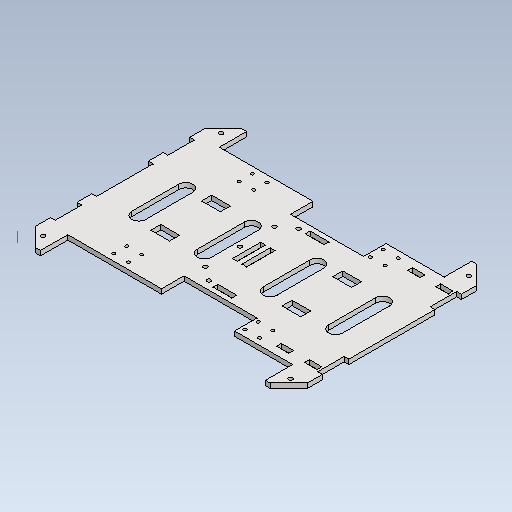
# Autodesk Inventor part: mid-plate
Saved by Autodesk Inventor 2025 (Build 290162000, 162)
## iProperties
Created: 2025-08-20
Part Number: mid-plate
Material: Generic
Document SubType Name: Modeling
Designer: HP
Density: 1 g/cm^3
Appearance: Default
Author: HP
Autodesk Inventor part; units mm, degrees
ref_plane "YZ Plane" through (0, 0, 0) normal (1, 0, 0) x (0, 1, 0)
ref_plane "XZ Plane" through (0, 0, 0) normal (0, 1, 0) x (-1, 0, 0)
ref_plane "XY Plane" through (0, 0, 0) normal (0, 0, 1) x (1, 0, 0)
sketch "Sketch1" plane through (0, 0, 0) normal (0, 1, 0) x (-1, 0, 0)
  line L0 (145, 110) -> (-145, 110)
  line L1 (-145, 110) -> (-145, -110)
  line L2 (-145, -110) -> (145, -110)
  line L3 (145, -110) -> (145, 110)
  line L4 (145, 110) -> (-145, -110) construction
  line L5 (-145, 110) -> (145, -110) construction
  line L6 (120, -80.8333) -> (20, -80.8333)
  line L7 (20, -80.8333) -> (20, -115.8333)
  line L8 (20, -115.8333) -> (120, -115.8333)
  line L9 (120, -115.8333) -> (120, -80.8333)
  line L10 (120, -80.8333) -> (20, -115.8333) construction
  line L11 (20, -80.8333) -> (120, -115.8333) construction
  line L12 (-20, -115.8333) -> (-120, -115.8333)
  line L13 (-120, -115.8333) -> (-120, -80.8333)
  line L14 (-120, -80.8333) -> (-20, -80.8333)
  line L15 (-20, -80.8333) -> (-20, -115.8333)
  line L16 (-20, -115.8333) -> (-120, -80.8333) construction
  line L17 (-120, -115.8333) -> (-20, -80.8333) construction
  line L18 (0, 110) -> (0, -110) construction
  point P0 (0, 0)
  point P1 (70, -98.3333)
  point P2 (-70, -98.3333)
  point P3 (0, 0)
  point P4 (-120, -110)
  point P5 (-20, -110)
  point P6 (120, -110)
  point P7 (20, -110)
  dimension "d1" = 100
  dimension "d2" = 100
  dimension "d3" = 35
  dimension "d4" = 35
  dimension "d5" = 140
  dimension "d6" = 11.6667
  dimension "d7" = 220
  dimension "d8" = 290
  constraints: 38 end point, 8 midpoint, 6 parallel, 3 horizontal, 3 perpendicular, 1 coincident, 1 horizontal alignment, 1 other
  measures "d1" distance between parallel lines of L7 L9
  measures "d2" distance between parallel lines of L13 L15
  measures "d3" distance between parallel lines of L6 L8
  measures "d4" distance between parallel lines of L14 L12
  measures "d5" distance of point (-70, -98.333) point (70, -98.333)
  measures "d6" distance from line of L2 point (70, -98.333)
  measures "d7" distance between parallel lines of L0 L2
  measures "d8" distance between parallel lines of L1 L3
extrude "Extrusion1" add sketch "Sketch1" along normal blind 5 contours L3 L2 L9 L6 L7 L15 L14 L13 L1 L0 | L2 L7 L6 L9 | L13 L14 L15 L2
extrude "Extrusion2" cut sketch "Sketch1" along normal blind 5 contours L9 L8 L7 L2 | L2 L7 L6 L9 | L13 L14 L15 L2
mirror "Mirror1" about plane through (0, 0, 0) normal (0, 0, 1) of "Extrusion2"
sketch "Sketch3" plane through (0, 5, 0) normal (0, 1, 0) x (1, 0, 0)
  line L0 (-120, -110) -> (-120, -80.8333) construction
  line L1 (-120, -80.8333) -> (-20, -80.8333) construction
  line L2 (-20, -80.8333) -> (-20, -110) construction
  line L3 (-20, -110) -> (20, -110) construction
  line L4 (20, -110) -> (20, -80.8333) construction
  line L5 (20, -80.8333) -> (120, -80.8333) construction
  line L6 (120, -80.8333) -> (120, -110) construction
  line L7 (120, -110) -> (145, -110) construction
  line L8 (145, -110) -> (145, 110) construction
  line L9 (145, 110) -> (120, 110) construction
  line L10 (120, 110) -> (120, 80.8333) construction
  line L11 (120, 80.8333) -> (20, 80.8333) construction
  line L12 (20, 80.8333) -> (20, 110) construction
  line L13 (20, 110) -> (-20, 110) construction
  line L14 (-20, 110) -> (-20, 80.8333) construction
  line L15 (-20, 80.8333) -> (-120, 80.8333) construction
  line L16 (-120, 80.8333) -> (-120, 110) construction
  line L17 (-120, 110) -> (-145, 110) projected
  line L18 (-145, 110) -> (-145, -110) construction
  line L19 (-145, -110) -> (-120, -110) construction
  circle A0 centre (-77.9, 73.7833) radius 1.6
  circle A1 centre (-62.1, 73.7833) radius 1.6
  circle A2 centre (-62.1, 59.8833) radius 1.6
  circle A3 centre (-77.9, 59.8833) radius 1.6
  line L20 (-77.9, 59.8833) -> (-62.1, 59.8833) construction
  line L21 (-62.1, 59.8833) -> (-62.1, 73.7833) construction
  line L22 (-62.1, 73.7833) -> (-77.9, 73.7833) construction
  line L23 (-77.9, 73.7833) -> (-77.9, 59.8833) construction
  line L24 (-77.9, 59.8833) -> (-62.1, 73.7833) construction
  line L25 (-62.1, 59.8833) -> (-77.9, 73.7833) construction
  point P0 (0, 0)
  point P1 (-70, 66.8333)
  point P2 (-70, 80.8333)
  dimension "d18" = 3.2
  dimension "d19" = 3.2
  dimension "d20" = 3.2
  dimension "d21" = 3.2
  dimension "d22" = 15.8
  dimension "d23" = 13.9
  dimension "d24" = 14
  constraints: 12 end point, 4 centre point, 4 coincident, 3 midpoint, 2 parallel, 1 horizontal, 1 perpendicular, 1 vertical alignment
  measures "d18" diameter of A0
  measures "d19" diameter of A1
  measures "d20" diameter of A3
  measures "d21" diameter of A2
  measures "d22" distance between parallel lines of L21 L23
  measures "d23" distance between parallel lines of L20 L22
  measures "d24" distance from line of point (-70, 66.833) L15
extrude "Extrusion4" cut sketch "Sketch3" against normal through all
mirror "Mirror4" about plane through (0, 0, 0) normal (1, 0, 0) of "Extrusion4"
mirror "Mirror5" about plane through (0, 0, 0) normal (0, 0, 1) of "Extrusion4", "Mirror4"
sketch "Sketch4" plane through (0, 5, 0) normal (0, 1, 0) x (1, 0, 0)
  circle A0 centre (62.1, -59.8833) radius 1.6 construction
  circle A1 centre (77.9, -59.8833) radius 1.6 construction
  circle A2 centre (62.1, -73.7833) radius 1.6 construction
  circle A3 centre (77.9, -73.7833) radius 1.6 construction
  circle A4 centre (-62.1, -59.8833) radius 1.6 construction
  circle A5 centre (-77.9, -59.8833) radius 1.6 construction
  circle A6 centre (-62.1, -73.7833) radius 1.6 construction
  circle A7 centre (-77.9, -73.7833) radius 1.6 construction
  circle A8 centre (62.1, 59.8833) radius 1.6 construction
  circle A9 centre (77.9, 59.8833) radius 1.6 construction
  circle A10 centre (62.1, 73.7833) radius 1.6 construction
  circle A11 centre (77.9, 73.7833) radius 1.6 construction
  circle A12 centre (-62.1, 59.8833) radius 1.6 construction
  circle A13 centre (-77.9, 73.7833) radius 1.6 construction
  circle A14 centre (-62.1, 73.7833) radius 1.6 construction
  circle A15 centre (-77.9, 59.8833) radius 1.6 construction
  line L0 (-120, -110) -> (-120, -80.8333) construction
  line L1 (-120, -80.8333) -> (-20, -80.8333) construction
  line L2 (-20, -80.8333) -> (-20, -110) construction
  line L3 (-20, -110) -> (20, -110) construction
  line L4 (20, -110) -> (20, -80.8333) construction
  line L5 (20, -80.8333) -> (120, -80.8333) construction
  line L6 (120, -80.8333) -> (120, -110) construction
  line L7 (120, -110) -> (145, -110) construction
  line L8 (145, -110) -> (145, 110) construction
  line L9 (145, 110) -> (120, 110) construction
  line L10 (120, 110) -> (120, 80.8333) construction
  line L11 (120, 80.8333) -> (20, 80.8333) construction
  line L12 (20, 80.8333) -> (20, 110) construction
  line L13 (20, 110) -> (-20, 110) construction
  line L14 (-20, 110) -> (-20, 80.8333) construction
  line L15 (-20, 80.8333) -> (-120, 80.8333) construction
  line L16 (-120, 80.8333) -> (-120, 110) construction
  line L17 (-120, 110) -> (-145, 110) construction
  line L18 (-145, 110) -> (-145, -110) construction
  line L19 (-145, -110) -> (-120, -110) construction
  line L20 (65, 17.6333) -> (45, 17.6333)
  line L21 (45, 17.6333) -> (45, 20.8333)
  line L22 (45, 20.8333) -> (65, 20.8333)
  line L23 (65, 20.8333) -> (65, 17.6333)
  line L24 (65, 17.6333) -> (45, 20.8333) construction
  line L25 (45, 17.6333) -> (65, 20.8333) construction
  point P0 (0, 0)
  point P1 (55, 19.2333)
  dimension "d27" = 20
  dimension "d28" = 3.2
  dimension "d29" = 80
  dimension "d30" = 60
  constraints: 12 end point, 2 midpoint, 2 parallel, 1 horizontal, 1 perpendicular
  measures "d27" distance between parallel lines of L23 L21
  measures "d28" distance between parallel lines of L22 L20
  measures "d29" distance between parallel lines of L8 L23
  measures "d30" distance between parallel lines of L11 L22
extrude "Extrusion5" [suppressed]
sketch "Sketch5" plane through (0, 5, 0) normal (0, 1, 0) x (1, 0, 0)
  circle A0 centre (62.1, -59.8833) radius 1.6 construction
  circle A1 centre (77.9, -59.8833) radius 1.6 construction
  circle A2 centre (62.1, -73.7833) radius 1.6 construction
  circle A3 centre (77.9, -73.7833) radius 1.6 construction
  circle A4 centre (-62.1, -59.8833) radius 1.6 construction
  circle A5 centre (-77.9, -59.8833) radius 1.6 construction
  circle A6 centre (-62.1, -73.7833) radius 1.6 construction
  circle A7 centre (-77.9, -73.7833) radius 1.6 construction
  circle A8 centre (62.1, 59.8833) radius 1.6 construction
  circle A9 centre (77.9, 59.8833) radius 1.6 construction
  circle A10 centre (62.1, 73.7833) radius 1.6 construction
  circle A11 centre (77.9, 73.7833) radius 1.6 construction
  circle A12 centre (-62.1, 59.8833) radius 1.6 construction
  circle A13 centre (-77.9, 73.7833) radius 1.6 construction
  circle A14 centre (-62.1, 73.7833) radius 1.6 construction
  circle A15 centre (-77.9, 59.8833) radius 1.6 construction
  line L0 (-120, -110) -> (-120, -80.8333) construction
  line L1 (-120, -80.8333) -> (-20, -80.8333) construction
  line L2 (-20, -80.8333) -> (-20, -110) projected
  line L3 (-20, -110) -> (20, -110) projected
  line L4 (20, -110) -> (20, -80.8333) projected
  line L5 (20, -80.8333) -> (120, -80.8333) construction
  line L6 (120, -80.8333) -> (120, -110) construction
  line L7 (120, -110) -> (145, -110) construction
  line L8 (145, -110) -> (145, 110) construction
  line L9 (145, 110) -> (120, 110) construction
  line L10 (120, 110) -> (120, 80.8333) construction
  line L11 (120, 80.8333) -> (20, 80.8333) construction
  line L12 (20, 80.8333) -> (20, 110) construction
  line L13 (20, 110) -> (-20, 110) construction
  line L14 (-20, 110) -> (-20, 80.8333) construction
  line L15 (-20, 80.8333) -> (-120, 80.8333) construction
  line L16 (-120, 80.8333) -> (-120, 110) construction
  line L17 (-120, 110) -> (-145, 110) construction
  line L18 (-145, 110) -> (-145, -110) construction
  line L19 (-145, -110) -> (-120, -110) construction
  line L20 (-20, -80.8333) -> (52, -80.8333)
  line L21 (52, -80.8333) -> (52, -56.8333)
  line L22 (52, -56.8333) -> (-20, -56.8333)
  line L23 (-20, -56.8333) -> (-20, -80.8333)
  line L24 (-20, -80.8333) -> (52, -56.8333) construction
  line L25 (52, -80.8333) -> (-20, -56.8333) construction
  line L26 (-20, -80.8333) -> (-20, -110) construction
  line L27 (124.4, -72.6) -> (137.6, -72.6)
  line L28 (137.6, -72.6) -> (137.6, -67.4)
  line L29 (137.6, -67.4) -> (124.4, -67.4)
  line L30 (124.4, -67.4) -> (124.4, -72.6)
  line L31 (124.4, -72.6) -> (137.6, -67.4) construction
  line L32 (137.6, -72.6) -> (124.4, -67.4) construction
  line L33 (26.1, -51.8333) -> (5.9, -51.8333)
  line L34 (5.9, -51.8333) -> (5.9, -46.6333)
  line L35 (5.9, -46.6333) -> (26.1, -46.6333)
  line L36 (26.1, -46.6333) -> (26.1, -51.8333)
  line L37 (26.1, -51.8333) -> (5.9, -46.6333) construction
  line L38 (5.9, -51.8333) -> (26.1, -46.6333) construction
  line L39 (60.2, -21.7333) -> (80.2, -21.7333)
  line L40 (80.2, -21.7333) -> (80.2, -32.4333)
  line L41 (80.2, -32.4333) -> (60.2, -32.4333)
  line L42 (60.2, -32.4333) -> (60.2, -21.7333)
  line L43 (60.2, -21.7333) -> (80.2, -32.4333) construction
  line L44 (80.2, -21.7333) -> (60.2, -32.4333) construction
  line L45 (-79.8, -32.4333) -> (-59.8, -32.4333)
  line L46 (-59.8, -32.4333) -> (-59.8, -21.7333)
  line L47 (-59.8, -21.7333) -> (-79.8, -21.7333)
  line L48 (-79.8, -21.7333) -> (-79.8, -32.4333)
  line L49 (-79.8, -32.4333) -> (-59.8, -21.7333) construction
  line L50 (-59.8, -32.4333) -> (-79.8, -21.7333) construction
  line L51 (52, -56.8333) -> (58, -56.8333)
  line L52 (58, -56.8333) -> (58, -80.8333)
  line L53 (58, -80.8333) -> (52, -80.8333)
  line L54 (52, -80.8333) -> (52, -56.8333)
  line L55 (94.4, -72.6) -> (107.6, -72.6)
  line L56 (107.6, -72.6) -> (107.6, -67.4)
  line L57 (107.6, -67.4) -> (94.4, -67.4)
  line L58 (94.4, -67.4) -> (94.4, -72.6)
  line L59 (94.4, -72.6) -> (107.6, -67.4) construction
  line L60 (107.6, -72.6) -> (94.4, -67.4) construction
  point P0 (0, 0)
  point P1 (16, -68.8333)
  point P2 (20, -80.8333)
  point P3 (131, -70)
  point P4 (131, -72.6)
  point P5 (16, -49.2333)
  point P6 (70.2, -27.0833)
  point P7 (-69.8, -27.0833)
  point P8 (52, -80.8333)
  point P9 (52, -80.8333)
  point P10 (101, -70)
  point P11 (101, -72.6)
  dimension "d33" = 24
  dimension "d34" = 72
  dimension "d37" = 13.2
  dimension "d38" = 5.2
  dimension "d40" = 14
  dimension "d55" = 20.2
  dimension "d56" = 5.2
  dimension "d57" = 5
  dimension "d60" = 20
  dimension "d61" = 10.7
  dimension "d62" = 53.75
  dimension "d63" = 74.8
  dimension "d64" = 75.2
  dimension "d65" = 10.7
  dimension "d66" = 20
  dimension "d85" = 6
  dimension "d105" = 70
  dimension "d106" = 13.2
  dimension "d107" = 5.2
  dimension "d108" = 30
  constraints: 80 end point, 14 midpoint, 14 parallel, 7 horizontal, 7 perpendicular, 2 collinear, 2 horizontal alignment, 1 point on line, 1 vertical alignment
  measures "d33" distance between parallel lines of L22 L20
  measures "d34" distance between parallel lines of L21 L23
  measures "d37" distance between parallel lines of L28 L30
  measures "d38" distance between parallel lines of L27 L29
  measures "d40" distance from line of L8 point (131, -72.6)
  measures "d55" distance of L34.end L35.end
  measures "d56" distance between parallel lines of L35 L33
  measures "d57" distance between parallel lines of L33 L22
  measures "d60" distance between parallel lines of L40 L42
  measures "d61" distance between parallel lines of L41 L39
  measures "d62" distance from line of point (70.2, -27.083) L5
  measures "d63" distance from line of L8 point (70.2, -27.083)
  measures "d64" distance from line of L18 point (-69.8, -27.083)
  measures "d65" distance between parallel lines of L45 L47
  measures "d66" distance between parallel lines of L46 L48
  measures "d85" distance between parallel lines of L52 L54
  measures "d105" vertical distance of point (131, -70) point (0, 0)
  measures "d106" distance between parallel lines of L56 L58
  measures "d107" distance between parallel lines of L55 L57
  measures "d108" distance of point (131, -70) point (101, -70)
extrude "Extrusion6" cut sketch "Sketch5" against normal through all
mirror "Mirror6" about plane through (0, 0, 0) normal (0, 0, 1) of "Extrusion6"
sketch "Sketch6" plane through (0, 5, 0) normal (0, 1, 0) x (1, 0, 0)
  circle A0 centre (-77.9, 59.8833) radius 1.6 construction
  circle A1 centre (-62.1, 73.7833) radius 1.6 construction
  circle A2 centre (-77.9, 73.7833) radius 1.6 construction
  circle A3 centre (-62.1, 59.8833) radius 1.6 construction
  circle A4 centre (77.9, 73.7833) radius 1.6 construction
  circle A5 centre (62.1, 73.7833) radius 1.6 construction
  circle A6 centre (77.9, 59.8833) radius 1.6 construction
  circle A7 centre (62.1, 59.8833) radius 1.6 construction
  circle A8 centre (-77.9, -73.7833) radius 1.6 construction
  circle A9 centre (-62.1, -73.7833) radius 1.6 construction
  circle A10 centre (-77.9, -59.8833) radius 1.6 construction
  circle A11 centre (-62.1, -59.8833) radius 1.6 construction
  circle A12 centre (77.9, -73.7833) radius 1.6 construction
  circle A13 centre (62.1, -73.7833) radius 1.6 construction
  circle A14 centre (77.9, -59.8833) radius 1.6 construction
  circle A15 centre (62.1, -59.8833) radius 1.6 construction
  line L0 (124.4, -67.4) -> (137.6, -67.4) construction
  line L1 (137.6, -67.4) -> (137.6, -72.6) construction
  line L2 (137.6, -72.6) -> (124.4, -72.6) construction
  line L3 (124.4, -72.6) -> (124.4, -67.4) construction
  line L4 (-20, 56.8333) -> (-20, 80.8333) construction
  line L5 (-20, 80.8333) -> (-120, 80.8333) construction
  line L6 (-120, 80.8333) -> (-120, 110) construction
  line L7 (-120, 110) -> (-145, 110) construction
  line L8 (-145, 110) -> (-145, -110) construction
  line L9 (-145, -110) -> (-120, -110) construction
  line L10 (-120, -110) -> (-120, -80.8333) construction
  line L11 (-120, -80.8333) -> (-20, -80.8333) construction
  line L12 (-20, -80.8333) -> (-20, -56.8333) construction
  line L13 (58, -80.8333) -> (120, -80.8333) construction
  line L14 (120, -80.8333) -> (120, -110) construction
  line L15 (120, -110) -> (145, -110) construction
  line L16 (145, -110) -> (145, 110) construction
  line L17 (145, 110) -> (120, 110) construction
  line L18 (120, 110) -> (120, 80.8333) construction
  line L19 (120, 80.8333) -> (58, 80.8333) construction
  line L20 (124.4, 67.4) -> (124.4, 72.6) construction
  line L21 (124.4, 72.6) -> (137.6, 72.6) construction
  line L22 (137.6, 72.6) -> (137.6, 67.4) construction
  line L23 (137.6, 67.4) -> (124.4, 67.4) construction
  line L24 (-140, 30.1) -> (-145, 30.1)
  line L25 (-145, 30.1) -> (-145, -30.1)
  line L26 (-145, -30.1) -> (-140, -30.1)
  line L27 (-140, -30.1) -> (-140, 30.1)
  line L28 (-140, 30.1) -> (-145, -30.1) construction
  line L29 (-145, 30.1) -> (-140, -30.1) construction
  line L30 (-145, 110) -> (-145, -110) projected
  line L31 (-10.1, 15.1) -> (-4.9, 15.1)
  line L32 (-4.9, 15.1) -> (-4.9, -15.1)
  line L33 (-4.9, -15.1) -> (-10.1, -15.1)
  line L34 (-10.1, -15.1) -> (-10.1, 15.1)
  line L35 (-10.1, 15.1) -> (-4.9, -15.1) construction
  line L36 (-4.9, 15.1) -> (-10.1, -15.1) construction
  line L37 (5.3, -15.1) -> (0.1, -15.1)
  line L38 (0.1, -15.1) -> (0.1, 15.1)
  line L39 (0.1, 15.1) -> (5.3, 15.1)
  line L40 (5.3, 15.1) -> (5.3, -15.1)
  line L41 (5.3, -15.1) -> (0.1, 15.1) construction
  line L42 (0.1, -15.1) -> (5.3, 15.1) construction
  line L43 (-100, 25) -> (-100, -25) construction
  line L44 (-107.5, 25) -> (-107.5, -25)
  line L45 (-92.5, -25) -> (-92.5, 25)
  arc A16 (-92.5, 25) -> (-107.5, 25) centre (-100, 25) ccw
  arc A17 (-107.5, -25) -> (-92.5, -25) centre (-100, -25) ccw
  line L46 (-30, 25) -> (-30, -25) construction
  line L47 (-37.5, 25) -> (-37.5, -25)
  line L48 (-22.5, -25) -> (-22.5, 25)
  arc A18 (-22.5, 25) -> (-37.5, 25) centre (-30, 25) ccw
  arc A19 (-37.5, -25) -> (-22.5, -25) centre (-30, -25) ccw
  line L49 (40, 25) -> (40, -25) construction
  line L50 (32.5, 25) -> (32.5, -25)
  line L51 (47.5, -25) -> (47.5, 25)
  arc A20 (47.5, 25) -> (32.5, 25) centre (40, 25) ccw
  arc A21 (32.5, -25) -> (47.5, -25) centre (40, -25) ccw
  line L52 (110, 25) -> (110, -25) construction
  line L53 (102.5, 25) -> (102.5, -25)
  line L54 (117.5, -25) -> (117.5, 25)
  arc A22 (117.5, 25) -> (102.5, 25) centre (110, 25) ccw
  arc A23 (102.5, -25) -> (117.5, -25) centre (110, -25) ccw
  line L55 (-20, -56.8333) -> (58, -56.8333) projected
  line L56 (58, -56.8333) -> (58, -80.8333) projected
  line L57 (58, 80.8333) -> (58, 56.8333) projected
  line L58 (58, 56.8333) -> (-20, 56.8333) projected
  point P0 (0, 0)
  point P1 (-142.5, 0)
  point P2 (-145, 0)
  point P3 (-7.5, 0)
  point P4 (2.7, 0)
  point P5 (-100, 0)
  point P6 (-30, 0)
  point P7 (40, 0)
  point P8 (110, 0)
  point P9 (-145, 0)
  dimension "d41" = 60.2
  dimension "d42" = 5
  dimension "d49" = 5.2
  dimension "d50" = 30.2
  dimension "d51" = 134.9
  dimension "d52" = 5.2
  dimension "d53" = 30.2
  dimension "d67" = 15
  dimension "d68" = 15
  dimension "d69" = 15
  dimension "d70" = 15
  dimension "d71" = 50
  dimension "d72" = 50
  dimension "d73" = 50
  dimension "d74" = 50
  dimension "d75" = 45
  dimension "d76" = 115
  dimension "d77" = 105
  dimension "d78" = 35
  dimension "d109" = 10.2
  constraints: 68 end point, 16 point on circle, 16 tangent, 13 parallel, 12 midpoint, 8 centre point, 7 horizontal alignment, 3 horizontal, 3 perpendicular, 1 collinear, 1 vertical
  measures "d41" distance between parallel lines of L26 L24
  measures "d42" distance between parallel lines of L8 L27
  measures "d49" distance of L32.end L33.end
  measures "d50" distance of L31.end L32.end
  measures "d51" distance between parallel lines of L8 L34
  measures "d52" distance between parallel lines of L38 L40
  measures "d53" distance between parallel lines of L39 L37
  measures "d67" distance between parallel lines of L51 L50
  measures "d68" distance between parallel lines of L45 L44
  measures "d69" distance between parallel lines of L48 L47
  measures "d70" distance between parallel lines of L54 L53
  measures "d71" distance of L52.start L52.end
  measures "d72" distance of L43.start L43.end
  measures "d73" distance of L46.start L46.end
  measures "d74" distance of L49.start L49.end
  measures "d75" distance from line of L8 point (-100, 0)
  measures "d76" distance from line of L8 point (-30, 0)
  measures "d77" distance from line of L16 point (40, 0)
  measures "d78" distance from line of L16 point (110, 0)
  measures "d109" distance of point (2.7, 0) point (-7.5, 0)
extrude "Extrusion7" cut sketch "Sketch6" against normal through all
chamfer "Chamfer1" distance 20 angle 45 4 edges at (-145, 2.5, 110) (-145, 2.5, -110) (145, 2.5, 110) (145, 2.5, -110)
sketch "Sketch8" plane through (0, 5, 0) normal (0, 1, 0) x (1, 0, 0)
  line L0 (125, 110) -> (145, 90) construction
  line L1 (125, 110) -> (120, 110) construction
  line L2 (120, 110) -> (120, 80.8333) construction
  line L3 (120, 80.8333) -> (58, 80.8333) construction
  line L4 (-20, 56.8333) -> (-20, 80.8333) construction
  line L5 (-20, 80.8333) -> (-120, 80.8333) construction
  line L6 (-120, 80.8333) -> (-120, 110) construction
  line L7 (-120, 110) -> (-125, 110) construction
  line L8 (-145, 90) -> (-125, 110) construction
  line L9 (-145, 90) -> (-145, 30.1) projected
  line L10 (-145, 30.1) -> (-140, 30.1) construction
  line L11 (-140, 30.1) -> (-140, -30.1) construction
  line L12 (-140, -30.1) -> (-145, -30.1) construction
  line L13 (-145, -30.1) -> (-145, -90) construction
  line L14 (-125, -110) -> (-145, -90) construction
  line L15 (-125, -110) -> (-120, -110) construction
  line L16 (-120, -110) -> (-120, -80.8333) construction
  line L17 (-120, -80.8333) -> (-20, -80.8333) construction
  line L18 (-20, -80.8333) -> (-20, -56.8333) construction
  line L19 (58, -80.8333) -> (120, -80.8333) construction
  line L20 (120, -80.8333) -> (120, -110) construction
  line L21 (120, -110) -> (125, -110) construction
  line L22 (145, -90) -> (125, -110) construction
  line L23 (145, -90) -> (145, 90) construction
  line L24 (124.4, -67.4) -> (137.6, -67.4) construction
  line L25 (137.6, -67.4) -> (137.6, -72.6) construction
  line L26 (137.6, -72.6) -> (124.4, -72.6) construction
  line L27 (124.4, -72.6) -> (124.4, -67.4) construction
  line L28 (5.9, -51.8333) -> (5.9, -46.6333) construction
  line L29 (5.9, -46.6333) -> (26.1, -46.6333) construction
  line L30 (26.1, -46.6333) -> (26.1, -51.8333) construction
  line L31 (26.1, -51.8333) -> (5.9, -51.8333) construction
  line L32 (80.2, -21.7333) -> (80.2, -32.4333) construction
  line L33 (80.2, -32.4333) -> (60.2, -32.4333) construction
  line L34 (60.2, -32.4333) -> (60.2, -21.7333) construction
  line L35 (60.2, -21.7333) -> (80.2, -21.7333) construction
  line L36 (-79.8, -21.7333) -> (-59.8, -21.7333) construction
  line L37 (-59.8, -21.7333) -> (-59.8, -32.4333) construction
  line L38 (-59.8, -32.4333) -> (-79.8, -32.4333) construction
  line L39 (-79.8, -32.4333) -> (-79.8, -21.7333) construction
  circle A0 centre (62.1, -59.8833) radius 1.6 construction
  circle A1 centre (77.9, -59.8833) radius 1.6 construction
  circle A2 centre (62.1, -73.7833) radius 1.6 construction
  circle A3 centre (77.9, -73.7833) radius 1.6 construction
  circle A4 centre (-62.1, -59.8833) radius 1.6 construction
  circle A5 centre (-77.9, -59.8833) radius 1.6 construction
  circle A6 centre (-62.1, -73.7833) radius 1.6 construction
  circle A7 centre (-77.9, -73.7833) radius 1.6 construction
  circle A8 centre (62.1, 59.8833) radius 1.6 construction
  circle A9 centre (77.9, 59.8833) radius 1.6 construction
  circle A10 centre (62.1, 73.7833) radius 1.6 construction
  circle A11 centre (77.9, 73.7833) radius 1.6 construction
  circle A12 centre (-62.1, 59.8833) radius 1.6 construction
  circle A13 centre (-77.9, 73.7833) radius 1.6 construction
  circle A14 centre (-62.1, 73.7833) radius 1.6 construction
  circle A15 centre (-77.9, 59.8833) radius 1.6 construction
  line L40 (26.1, 51.8333) -> (26.1, 46.6333) construction
  line L41 (26.1, 46.6333) -> (5.9, 46.6333) construction
  line L42 (5.9, 46.6333) -> (5.9, 51.8333) construction
  line L43 (5.9, 51.8333) -> (26.1, 51.8333) construction
  line L44 (80.2, 21.7333) -> (60.2, 21.7333) construction
  line L45 (60.2, 21.7333) -> (60.2, 32.4333) construction
  line L46 (60.2, 32.4333) -> (80.2, 32.4333) construction
  line L47 (80.2, 32.4333) -> (80.2, 21.7333) construction
  line L48 (-79.8, 32.4333) -> (-59.8, 32.4333) construction
  line L49 (-59.8, 32.4333) -> (-59.8, 21.7333) construction
  line L50 (-59.8, 21.7333) -> (-79.8, 21.7333) construction
  line L51 (-79.8, 21.7333) -> (-79.8, 32.4333) construction
  line L52 (124.4, 72.6) -> (137.6, 72.6) construction
  line L53 (137.6, 72.6) -> (137.6, 67.4) construction
  line L54 (137.6, 67.4) -> (124.4, 67.4) construction
  line L55 (124.4, 67.4) -> (124.4, 72.6) construction
  line L56 (-4.9, 15.1) -> (-4.9, -15.1) construction
  line L57 (-4.9, -15.1) -> (-10.1, -15.1) construction
  line L58 (-10.1, -15.1) -> (-10.1, 15.1) construction
  line L59 (-10.1, 15.1) -> (-4.9, 15.1) construction
  line L60 (-22.5, 25) -> (-22.5, -25) construction
  arc A16 (-37.5, -25) -> (-22.5, -25) centre (-30, -25) ccw construction
  line L61 (-37.5, -25) -> (-37.5, 25) construction
  arc A17 (-22.5, 25) -> (-37.5, 25) centre (-30, 25) ccw construction
  line L62 (-92.5, 25) -> (-92.5, -25) construction
  arc A18 (-107.5, -25) -> (-92.5, -25) centre (-100, -25) ccw construction
  line L63 (-107.5, -25) -> (-107.5, 25) construction
  arc A19 (-92.5, 25) -> (-107.5, 25) centre (-100, 25) ccw construction
  line L64 (117.5, 25) -> (117.5, -25) construction
  arc A20 (102.5, -25) -> (117.5, -25) centre (110, -25) ccw construction
  line L65 (102.5, -25) -> (102.5, 25) construction
  arc A21 (117.5, 25) -> (102.5, 25) centre (110, 25) ccw construction
  line L66 (0.1, -15.1) -> (0.1, 15.1) construction
  line L67 (0.1, 15.1) -> (5.3, 15.1) construction
  line L68 (5.3, 15.1) -> (5.3, -15.1) construction
  line L69 (5.3, -15.1) -> (0.1, -15.1) construction
  line L70 (47.5, 25) -> (47.5, -25) construction
  arc A22 (32.5, -25) -> (47.5, -25) centre (40, -25) ccw construction
  line L71 (32.5, -25) -> (32.5, 25) construction
  arc A23 (47.5, 25) -> (32.5, 25) centre (40, 25) ccw construction
  circle A24 centre (-2.4, -48) radius 2.1
  line L72 (-4.9, -15.1) -> (0.1, -15.1) construction
  circle A25 centre (-2.4, 48) radius 2.1
  line L73 (58, 80.8333) -> (58, 56.8333) projected
  line L74 (58, 56.8333) -> (-20, 56.8333) projected
  line L75 (-20, -56.8333) -> (58, -56.8333) projected
  line L76 (58, -56.8333) -> (58, -80.8333) projected
  line L77 (-145, 45.95) -> (-140, 45.95)
  line L78 (-140, 45.95) -> (-140, 74.15)
  line L79 (-140, 74.15) -> (-145, 74.15)
  line L80 (-145, 74.15) -> (-145, 45.95)
  line L81 (-145, 45.95) -> (-140, 74.15) construction
  line L82 (-140, 45.95) -> (-145, 74.15) construction
  line L83 (-145, 90) -> (-145, 30.1) projected
  line L84 (-145, -45.95) -> (-140, -45.95)
  line L85 (-140, -45.95) -> (-140, -74.15)
  line L86 (-140, -74.15) -> (-145, -74.15)
  line L87 (-145, -74.15) -> (-145, -45.95)
  line L88 (-145, -45.95) -> (-140, -74.15) construction
  line L89 (-140, -45.95) -> (-145, -74.15) construction
  line L90 (140, 74.15) -> (145, 74.15)
  line L91 (145, 74.15) -> (145, 45.95)
  line L92 (145, 45.95) -> (140, 45.95)
  line L93 (140, 45.95) -> (140, 74.15)
  line L94 (140, 74.15) -> (145, 45.95) construction
  line L95 (145, 74.15) -> (140, 45.95) construction
  line L96 (140, -45.95) -> (145, -45.95)
  line L97 (145, -45.95) -> (145, -74.15)
  line L98 (145, -74.15) -> (140, -74.15)
  line L99 (140, -74.15) -> (140, -45.95)
  line L100 (140, -45.95) -> (145, -74.15) construction
  line L101 (145, -45.95) -> (140, -74.15) construction
  line L102 (145, -90) -> (145, 90) construction
  circle A26 centre (-17.1, -37) radius 2.1
  circle A27 centre (-17.1, 0) radius 2.1
  circle A28 centre (-17.1, 37) radius 2.1
  point P0 (0, 0)
  point P1 (-2.4, -15.1)
  point P2 (-142.5, 60.05)
  point P3 (-145, 60.05)
  point P4 (-142.5, -60.05)
  point P5 (-145, -60.05)
  point P6 (142.5, 60.05)
  point P7 (142.5, -60.05)
  point P8 (0.1, 0)
  dimension "d79" = 4.2
  dimension "d80" = 4.2
  dimension "d88" = 5
  dimension "d89" = 28.2
  dimension "d91" = 28.2
  dimension "d92" = 5
  dimension "d93" = 28.2
  dimension "d94" = 28.2
  dimension "d95" = 5
  dimension "d96" = 5
  dimension "d110" = 4.2
  dimension "d111" = 4.2
  dimension "d112" = 4.2
  dimension "d113" = 37
  dimension "d114" = 37
  dimension "d115" = 7
  dimension "d116" = 48
  dimension "d117" = 48
  constraints: 50 end point, 12 midpoint, 8 parallel, 5 centre point, 5 horizontal, 5 horizontal alignment, 5 vertical alignment, 4 perpendicular, 3 collinear
  measures "d79" diameter of A24
  measures "d80" diameter of A25
  measures "d88" distance between parallel lines of L80 L78
  measures "d89" distance between parallel lines of L77 L79
  measures "d91" distance between parallel lines of L86 L84
  measures "d92" distance between parallel lines of L87 L85
  measures "d93" distance between parallel lines of L98 L96
  measures "d94" distance between parallel lines of L92 L90
  measures "d95" distance between parallel lines of L91 L93
  measures "d96" distance between parallel lines of L23 L99
  measures "d110" diameter of A26
  measures "d111" diameter of A27
  measures "d112" diameter of A28
  measures "d113" distance of A27.centre A28.centre
  measures "d114" distance of A26.centre A27.centre
  measures "d115" distance from line of A27.centre L58
  measures "d116" vertical distance of point (0, 0) A25.centre
  measures "d117" vertical distance of A24.centre point (0, 0)
extrude "Extrusion8" cut sketch "Sketch8" against normal through all
sketch "Sketch9" plane through (0, 5, 0) normal (0, 1, 0) x (1, 0, 0)
  line L0 (47.5, 25) -> (47.5, -25) construction
  arc A0 (32.5, -25) -> (47.5, -25) centre (40, -25) ccw construction
  line L1 (32.5, -25) -> (32.5, 25) construction
  arc A1 (47.5, 25) -> (32.5, 25) centre (40, 25) ccw construction
  line L2 (0.1, -15.1) -> (0.1, 15.1) construction
  line L3 (0.1, 15.1) -> (5.3, 15.1) construction
  line L4 (5.3, 15.1) -> (5.3, -15.1) construction
  line L5 (5.3, -15.1) -> (0.1, -15.1) construction
  line L6 (117.5, 25) -> (117.5, -25) construction
  arc A2 (102.5, -25) -> (117.5, -25) centre (110, -25) ccw construction
  line L7 (102.5, -25) -> (102.5, 25) construction
  arc A3 (117.5, 25) -> (102.5, 25) centre (110, 25) ccw construction
  line L8 (-92.5, 25) -> (-92.5, -25) construction
  arc A4 (-107.5, -25) -> (-92.5, -25) centre (-100, -25) ccw construction
  line L9 (-107.5, -25) -> (-107.5, 25) construction
  arc A5 (-92.5, 25) -> (-107.5, 25) centre (-100, 25) ccw construction
  line L10 (-22.5, 25) -> (-22.5, -25) construction
  arc A6 (-37.5, -25) -> (-22.5, -25) centre (-30, -25) ccw construction
  line L11 (-37.5, -25) -> (-37.5, 25) construction
  arc A7 (-22.5, 25) -> (-37.5, 25) centre (-30, 25) ccw construction
  line L12 (-4.9, 15.1) -> (-4.9, -15.1) construction
  line L13 (-4.9, -15.1) -> (-10.1, -15.1) construction
  line L14 (-10.1, -15.1) -> (-10.1, 15.1) construction
  line L15 (-10.1, 15.1) -> (-4.9, 15.1) construction
  line L16 (26.1, 51.8333) -> (26.1, 46.6333) construction
  line L17 (26.1, 46.6333) -> (5.9, 46.6333) construction
  line L18 (5.9, 46.6333) -> (5.9, 51.8333) construction
  line L19 (5.9, 51.8333) -> (26.1, 51.8333) construction
  line L20 (60.2, 21.7333) -> (60.2, 32.4333) construction
  line L21 (60.2, 32.4333) -> (80.2, 32.4333) construction
  line L22 (80.2, 32.4333) -> (80.2, 21.7333) construction
  line L23 (80.2, 21.7333) -> (60.2, 21.7333) construction
  line L24 (-79.8, 21.7333) -> (-79.8, 32.4333) construction
  line L25 (-79.8, 32.4333) -> (-59.8, 32.4333) construction
  line L26 (-59.8, 32.4333) -> (-59.8, 21.7333) construction
  line L27 (-59.8, 21.7333) -> (-79.8, 21.7333) construction
  line L28 (124.4, 72.6) -> (137.6, 72.6) construction
  line L29 (137.6, 72.6) -> (137.6, 67.4) construction
  line L30 (137.6, 67.4) -> (124.4, 67.4) construction
  line L31 (124.4, 67.4) -> (124.4, 72.6) construction
  circle A8 centre (-77.9, 59.8833) radius 1.6 construction
  circle A9 centre (-62.1, 73.7833) radius 1.6 construction
  circle A10 centre (-77.9, 73.7833) radius 1.6 construction
  circle A11 centre (-62.1, 59.8833) radius 1.6 construction
  circle A12 centre (77.9, 73.7833) radius 1.6 construction
  circle A13 centre (62.1, 73.7833) radius 1.6 construction
  circle A14 centre (77.9, 59.8833) radius 1.6 construction
  circle A15 centre (62.1, 59.8833) radius 1.6 construction
  circle A16 centre (-77.9, -73.7833) radius 1.6 construction
  circle A17 centre (-62.1, -73.7833) radius 1.6 construction
  circle A18 centre (-77.9, -59.8833) radius 1.6 construction
  circle A19 centre (-62.1, -59.8833) radius 1.6 construction
  circle A20 centre (77.9, -73.7833) radius 1.6 construction
  circle A21 centre (62.1, -73.7833) radius 1.6 construction
  circle A22 centre (77.9, -59.8833) radius 1.6 construction
  circle A23 centre (62.1, -59.8833) radius 1.6 construction
  line L32 (80.2, -21.7333) -> (80.2, -32.4333) construction
  line L33 (80.2, -32.4333) -> (60.2, -32.4333) construction
  line L34 (60.2, -32.4333) -> (60.2, -21.7333) construction
  line L35 (60.2, -21.7333) -> (80.2, -21.7333) construction
  line L36 (-79.8, -21.7333) -> (-59.8, -21.7333) construction
  line L37 (-59.8, -21.7333) -> (-59.8, -32.4333) construction
  line L38 (-59.8, -32.4333) -> (-79.8, -32.4333) construction
  line L39 (-79.8, -32.4333) -> (-79.8, -21.7333) construction
  line L40 (124.4, -67.4) -> (137.6, -67.4) construction
  line L41 (137.6, -67.4) -> (137.6, -72.6) construction
  line L42 (137.6, -72.6) -> (124.4, -72.6) construction
  line L43 (124.4, -72.6) -> (124.4, -67.4) construction
  line L44 (5.9, -51.8333) -> (5.9, -46.6333) construction
  line L45 (5.9, -46.6333) -> (26.1, -46.6333) construction
  line L46 (26.1, -46.6333) -> (26.1, -51.8333) construction
  line L47 (26.1, -51.8333) -> (5.9, -51.8333) construction
  circle A24 centre (-2.4, 48) radius 2.1 construction
  circle A25 centre (-2.4, -48) radius 2.1 construction
  line L48 (-145, 74.15) -> (-140, 74.15) construction
  line L49 (-140, 74.15) -> (-140, 45.95) construction
  line L50 (-140, 45.95) -> (-145, 45.95) construction
  line L51 (-145, 45.95) -> (-145, 30.1) construction
  line L52 (-145, 30.1) -> (-140, 30.1) construction
  line L53 (-140, 30.1) -> (-140, -30.1) construction
  line L54 (-140, -30.1) -> (-145, -30.1) construction
  line L55 (-145, -30.1) -> (-145, -45.95) construction
  line L56 (-145, -45.95) -> (-140, -45.95) construction
  line L57 (-140, -45.95) -> (-140, -74.15) construction
  line L58 (-140, -74.15) -> (-145, -74.15) construction
  line L59 (-145, -74.15) -> (-145, -90) construction
  line L60 (-125, -110) -> (-145, -90) construction
  line L61 (-125, -110) -> (-120, -110) construction
  line L62 (-120, -110) -> (-120, -80.8333) construction
  line L63 (-120, -80.8333) -> (-20, -80.8333) construction
  line L64 (-20, -80.8333) -> (-20, -56.8333) construction
  line L65 (-20, -56.8333) -> (58, -56.8333) construction
  line L66 (58, -56.8333) -> (58, -80.8333) construction
  line L67 (58, -80.8333) -> (120, -80.8333) construction
  line L68 (120, -80.8333) -> (120, -110) construction
  line L69 (120, -110) -> (125, -110) construction
  line L70 (145, -90) -> (125, -110) construction
  line L71 (145, -90) -> (145, -74.15) construction
  line L72 (145, -74.15) -> (140, -74.15) construction
  line L73 (140, -74.15) -> (140, -45.95) construction
  line L74 (140, -45.95) -> (145, -45.95) construction
  line L75 (145, -45.95) -> (145, 45.95) construction
  line L76 (145, 45.95) -> (140, 45.95) construction
  line L77 (140, 45.95) -> (140, 74.15) construction
  line L78 (140, 74.15) -> (145, 74.15) construction
  line L79 (145, 74.15) -> (145, 90) construction
  line L80 (125, 110) -> (145, 90) construction
  line L81 (125, 110) -> (120, 110) construction
  line L82 (120, 110) -> (120, 80.8333) construction
  line L83 (120, 80.8333) -> (58, 80.8333) construction
  line L84 (58, 80.8333) -> (58, 56.8333) construction
  line L85 (58, 56.8333) -> (-20, 56.8333) construction
  line L86 (-20, 56.8333) -> (-20, 80.8333) construction
  line L87 (-20, 80.8333) -> (-120, 80.8333) construction
  line L88 (-120, 80.8333) -> (-120, 110) construction
  line L89 (-120, 110) -> (-125, 110) construction
  line L90 (-145, 90) -> (-125, 110) construction
  line L91 (-145, 90) -> (-145, 74.15) construction
  circle A26 centre (-132, -95) radius 2.1
  circle A27 centre (132, -95) radius 2.1
  point P0 (0, 0)
  dimension "d97" = 4.2
  dimension "d98" = 4.2
  dimension "d99" = 13
  dimension "d100" = 13
  dimension "d101" = 5
  dimension "d102" = 5
  constraints: 2 centre point
  measures "d97" diameter of A26
  measures "d98" diameter of A27
  measures "d99" distance from line of L71 A27.centre
  measures "d100" distance from line of L59 A26.centre
  measures "d101" vertical distance of A26.centre L59.end
  measures "d102" vertical distance of L70.start A27.centre
extrude "Extrusion9" cut sketch "Sketch9" against normal through all
mirror "Mirror7" about plane through (0, 0, 0) normal (0, 0, 1) of "Extrusion9"
equation "\"d2\" = d1"
equation "\"d4\" = d3"
equation "\"d6\" = 0.333333 * d3"
equation "\"d19\" = d18"
equation "\"d20\" = d18"
equation "\"d21\" = d18"
equation "\"d65\" = d61"
equation "\"d66\" = d60"
equation "\"d67\" = d68"
equation "\"d69\" = d68"
equation "\"d70\" = d67"
equation "\"d71\" = d74"
equation "\"d73\" = d72"
equation "\"d74\" = d73"
body "Solid1"
